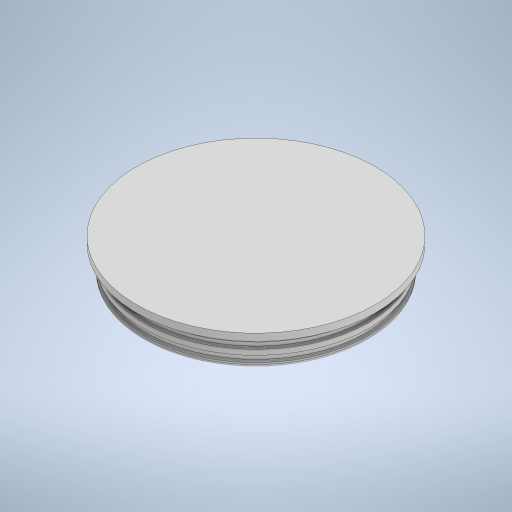
# Autodesk Inventor part: Rebreather-Endcap-Insert
Saved by Autodesk Inventor 2023 (Build 270158000, 158)
## iProperties
Created: 2022-11-09
Part Number: Rebreather-Endcap-Insert
Material: Generic
Document SubType Name: Modeling
Designer: incep
Density: 1 g/cm^3
Appearance: Default
Author: incep
## iProperties of the stored document Rebreather-Endcap-Insert_3DPrint.ipt
Created: 2022-11-09
Part Number: Rebreather-Endcap-Insert_3DPrint
Material: Generic
Document SubType Name: Modeling
Designer: incep
Density: 1 g/cm^3
Appearance: Default
Author: incep
Autodesk Inventor part; units mm, degrees
ref_plane "YZ Plane" through (0, 0, 0) normal (1, 0, 0) x (0, 1, 0)
ref_plane "XZ Plane" through (0, 0, 0) normal (0, 1, 0) x (-1, 0, 0)
ref_plane "XY Plane" through (0, 0, 0) normal (0, 0, 1) x (1, 0, 0)
sketch "Sketch1" plane through (0, 0, 0) normal (0, 0, 1) x (1, 0, 0)
  line L0 (-63.75, 0) -> (63.75, 0) construction
  line L1 (63.75, 0) -> (63.75, -15.9)
  line L2 (63.75, -15.9) -> (-63.75, -15.9)
  line L3 (-63.75, -15.9) -> (-63.75, 0)
  line L4 (61.63, -2.97) -> (63.75, -2.97)
  line L5 (63.75, -2.97) -> (63.75, -6.47)
  line L6 (63.75, -6.47) -> (61.63, -6.47)
  line L7 (61.63, -6.47) -> (61.63, -2.97)
  line L8 (61.63, -9.44) -> (63.75, -9.44)
  line L9 (63.75, -9.44) -> (63.75, -12.94)
  line L10 (63.75, -12.94) -> (61.63, -12.94)
  line L11 (61.63, -12.94) -> (61.63, -9.44)
  line L12 (-57.63, 0) -> (57.63, 0)
  line L13 (57.63, 0) -> (57.63, -15.9)
  line L14 (57.63, -15.9) -> (-57.63, -15.9)
  line L15 (-57.63, -15.9) -> (-57.63, 0)
  line L16 (-67.45, 4) -> (67.45, 4)
  line L17 (67.45, 4) -> (67.45, 0)
  line L18 (67.45, 0) -> (-67.45, 0) construction
  line L19 (-67.45, 0) -> (-67.45, 4)
  line L20 (63.75, 0) -> (67.45, 0)
  line L21 (0, 0) -> (0, 4)
  point P0 (61.63, -11.19)
  dimension "d0" = 127.5
  dimension "d1" = 15.9
  dimension "d2" = 3.5
  dimension "d4" = 3.5
  dimension "d6" = 2.97
  dimension "d7" = 2.97
  dimension "d8" = 134.9
  dimension "d9" = 4
  dimension "d10" = 4
  dimension "d11" = 61.63
  dimension "d12" = 2.12
  constraints: 44 end point, 10 parallel, 7 collinear, 5 horizontal, 5 midpoint, 5 perpendicular, 4 coincident
  measures "d0" distance of L0.start L0.end
  measures "d1" distance of L2.end L0.start
  measures "d2" distance of L6.end L4.start
  measures "d4" distance of L10.end L8.start
  measures "d6" distance between parallel lines of L0 L4
  measures "d7" distance between parallel lines of L8 L6
  measures "d8" distance of L16.start L16.end
  measures "d9" distance between parallel lines of L18 L16
  measures "d10" distance from line of point (61.63, -11.19) L13
  measures "d11" distance from line of L7 point (0, 0)
  measures "d12" distance of L4.start L4.end
revolve "Revolution1" add sketch "Sketch1" angle 360 about axis through (0, 0, 0) along (0, 1, 0) contours L1 L4 L7 L6 L8 L11 L10 L2 L13 L12 L21 L16 L17 L20
sketch "Sketch2" plane through (0, 0, 0) normal (0, -1, 0) x (1, 0, 0)
  line L0 (-58.5, 2) -> (58.5, 2)
  line L1 (58.5, 2) -> (58.5, -2)
  line L2 (58.5, -2) -> (-58.5, -2)
  line L3 (-58.5, -2) -> (-58.5, 2)
  circle A0 centre (0, 0) radius 57.63 projected
  circle A1 centre (0, 0) radius 63.75 projected
  point P0 (58.5, 0)
  point P1 (0, 2)
  point P2 (57.5953, 2)
  point P3 (-57.5953, 2)
  point P4 (-57.5953, -2)
  point P5 (57.5953, -2)
  dimension "d14" = 4
  dimension "d15" = 117
  constraints: 8 end point, 2 midpoint, 2 parallel, 1 horizontal, 1 horizontal alignment, 1 perpendicular, 1 vertical alignment
  measures "d14" distance between parallel lines of L2 L0
  measures "d15" distance of L0.start L0.end
extrude "Extrusion1" add sketch "Sketch2" along normal blind 7.5 contours L0 A0 L2
pattern_circular "Circular Pattern1" count 3 over 360 about axis through (0, -10, 0) along (0, 1, 0) of "Extrusion1"
fillet "Fillet1" radius 2 39 edges at (-63.75, -15.9, 0) (-57.63, -15.9, 0) (30.5297, 0, -2) (30.5297, 0, 2) (16.9969, 0, 25.4395) (13.5328, 0, 27.4395) (-13.5328, 0, 27.4395) (16.9969, 0, -25.4395) (-16.9969, 0, 25.4395) (13.5328, 0, -27.4395) (-16.9969, 0, -25.4395) (-30.5297, 0, -2) (-30.5297, 0, 2) (-13.5328, 0, -27.4395) (49.909, 0, 28.815) (0, 0, 57.63) (49.909, 0, -28.815) (-49.909, 0, 28.815) (0, 0, -57.63) (-49.909, 0, -28.815) (27.0656, -3.75, 50.879) (30.5297, -3.75, 48.879) (28.815, -7.5, 49.909) (57.5953, -3.75, 2) (57.6213, -7.5, -1.0002) (57.6213, -7.5, 1.0002) (57.5953, -3.75, -2) (-28.815, -7.5, 49.909) (-30.5297, -3.75, 48.879) (-27.0656, -3.75, 50.879) (-57.5953, -3.75, -2) (-57.63, -7.5, 0) (-57.5953, -3.75, 2) (-28.815, -7.5, -49.909) (-27.0656, -3.75, -50.879) (-30.5297, -3.75, -48.879) (27.0656, -3.75, -50.879) (28.815, -7.5, -49.909) (30.5297, -3.75, -48.879)
body "Solid1"
